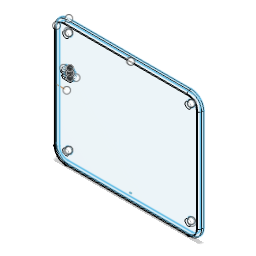
Logger transparent top v11 (Autodesk Fusion 360 design; units mm, degrees)
Autodesk Fusion 360 part; units mm, degrees
sketch "Sketch1" plane through (0, 0, 0) normal (0, 0, 1) x (1, 0, 0)
  arc A0 (29.5, -30.5) -> (35.5, -24.5) centre (29.5, -24.5) ccw
  arc A1 (35.5, 24.5) -> (29.5, 30.5) centre (29.5, 24.5) ccw
  circle A2 centre (29.5, 24.5) radius 1.5
  line L0 (-35.5, 24.5) -> (-35.5, -24.5)
  line L1 (29.5, -30.5) -> (-29.5, -30.5)
  line L2 (-29.5, 30.5) -> (29.5, 30.5)
  arc A3 (34, 25) -> (30, 29) centre (30, 25) ccw
  circle A4 centre (29.5, -24.5) radius 1.5
  arc A5 (30, -29) -> (34, -25) centre (30, -25) ccw
  line L3 (30, -29) -> (-30, -29)
  arc A6 (-34, -25) -> (-30, -29) centre (-30, -25) ccw
  line L4 (0, -27.5) -> (0.5, -27.5) construction
  arc A7 (-35.5, -24.5) -> (-29.5, -30.5) centre (-29.5, -24.5) ccw
  line L5 (-30, 29) -> (30, 29)
  arc A8 (-29.5, 30.5) -> (-35.5, 24.5) centre (-29.5, 24.5) ccw
  line L6 (0, 27.5) -> (0.5, 27.5) construction
  circle A9 centre (-29.5, 24.5) radius 1.5
  arc A10 (-30, 29) -> (-34, 25) centre (-30, 25) ccw
  line L7 (0, -27.5) -> (0.5, -27.5) construction
  line L8 (-34, -25) -> (-34, 25)
  circle A11 centre (-29.5, -24.5) radius 1.5
  line L9 (0, -27.5) -> (0.5, -27.5)
  arc A12 (-29.5, 30.5) -> (-35.5, 24.5) centre (-29.5, 24.5) ccw
  line L10 (34, 25) -> (34, -25)
  line L11 (35.5, 24.5) -> (35.5, -24.5)
  line L12 (-35.5, 0) -> (-30.5, 0) construction
  line L13 (-29, 8.5) -> (-29, 9.5) construction
  line L14 (-26.042, 8.5) -> (-31.958, 8.5)
  line L15 (-31.958, 7.5) -> (-26.042, 7.5)
  line L16 (-29, 8.5) -> (-29, 10) construction
  line L17 (-27.3417, 10.5) -> (-30.6583, 10.5)
  line L18 (-31.5981, 9.5) -> (-26.4019, 9.5)
  line L19 (-29, 7.5) -> (-29, 6) construction
  arc A13 (-30.6583, 10.5) -> (-31.5981, 9.5) centre (-29, 8) ccw
  arc A14 (-26.4019, 9.5) -> (-27.3417, 10.5) centre (-29, 8) ccw
  line L20 (-32, 8.5) -> (-31.9592, 8.4932) construction
  line L21 (-26.0408, 7.5068) -> (-26, 7.5) construction
  line L22 (-26.4019, 6.5) -> (-31.5981, 6.5)
  line L23 (-30.6583, 5.5) -> (-27.3417, 5.5)
  arc A15 (-31.958, 8.5) -> (-31.958, 7.5) centre (-29, 8) ccw
  arc A16 (-26.042, 7.5) -> (-26.042, 8.5) centre (-29, 8) ccw
  arc A17 (-31.5981, 6.5) -> (-30.6583, 5.5) centre (-29, 8) ccw
  arc A18 (-27.3417, 5.5) -> (-26.4019, 6.5) centre (-29, 8) ccw
  point P0 (-29, 8)
  point P1 (-29, 8)
  point P2 (-29, 10)
  point P3 (-29, 6)
  point P4 (-29, 6)
  dimension "d1" = 3
  dimension "d2" = 3
  dimension "d3" = 3
  dimension "d4" = 3
  dimension "d25" = 1.5
  constraint horizontal L3
  constraint perpendicular L3 L8
  constraint parallel L3 L5
  constraint parallel L8 L10
  constraint tangent L5 A10
  constraint tangent A10 L8
  constraint tangent A1 L2
  constraint tangent A0 L11
  constraint tangent L1 A7
  constraint tangent L0 A7
  constraint midpoint L0 L12.start
  constraint perpendicular L8 L12
  constraint coincident P1 P0
  constraint horizontal L14
  constraint parallel L14 L15
  constraint coincident P1 L20
  constraint horizontal L17
  constraint parallel L17 L18
  constraint coincident P2 L16.end
  constraint perpendicular L15 L19
  constraint coincident P4 P3
  constraint concentric A13 A15
  constraint coincident L18.end A15
  constraint concentric A14 A15
  constraint coincident L15.end A15
  constraint coincident L15 L19.start
  constraint coincident L21.start A15
  constraint collinear L20 L21
  constraint coincident L20.end A15
  constraint horizontal L22
  constraint parallel L22 L23
  constraint concentric A15 A17
  constraint concentric A16 A17
  constraint coincident L23.end A17
  constraint concentric A17 A18
  measures "d1" diameter of A9
  measures "d2" diameter of A2
  measures "d3" diameter of A4
  measures "d4" diameter of A11
  measures "d25" distance of L13.start P2
extrude "Extrude3" add sketch "Sketch1" along normal blind 2 contours A0 A1 L0 L1 L2 A7 A8 A12 L11
fillet "Fillet1" radius 1 8 edges at (-33.7426, 28.7426, 2) (-35.5, 0, 2) (-33.7426, -28.7426, 2) (0, -30.5, 2) (33.7426, -28.7426, 2) (35.5, 0, 2) (33.7426, 28.7426, 2) (0, 30.5, 2)
extrude "Extrude4" add sketch "Sketch1" along normal blind 1.5 contours A3 A5 L3 A6 L5 A10 L8 L10
extrude "Extrude2" [suppressed]
